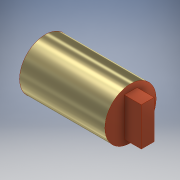
# Autodesk Inventor part: 레이져
Saved by Autodesk Inventor 2018 (Build 220112000, 112)
## iProperties
Created: 2018-04-19
Part Number: 레이져
Material: 일반
Document SubType Name: Modeling
Designer: CK
Density: 1 g/cm^3
Appearance: 금속 1400F 열
Author: CK
Autodesk Inventor part; units mm, degrees
ref_plane "YZ Plane" through (0, 0, 0) normal (1, 0, 0) x (0, 1, 0)
ref_plane "XZ Plane" through (0, 0, 0) normal (0, 1, 0) x (-1, 0, 0)
ref_plane "XY Plane" through (0, 0, 0) normal (0, 0, 1) x (1, 0, 0)
sketch "스케치1" plane through (0, 0, 0) normal (1, 0, 0) x (0, 1, 0)
  circle A0 centre (0, 0) radius 3
  dimension "d0" = 6
  constraints: 1 centre point, 1 coincident
  measures "d0" diameter of A0
extrude "돌출1" add sketch "스케치1" along normal blind 10
sketch "스케치2" plane through (0, 0, 0) normal (-1, 0, 0) x (0, 0, 1)
  circle A0 centre (0, 0) radius 1.5
  dimension "d3" = 3
  constraints: 1 centre point, 1 coincident
  measures "d3" diameter of A0
extrude "돌출2" cut sketch "스케치2" against normal blind 9
sketch "스케치4" plane through (0, 0, 0) normal (-1, 0, 0) x (0, 0, 1)
  arc A0 (-1.5, 0) -> (1.5, 0) centre (0, 0) ccw
  line L0 (-1.5, 0) -> (1.5, 0)
  line L1 (-2.0992, 0) -> (3.7582, 0)
  constraints: 4 end point, 2 horizontal, 2 point on circle, 1 centre point, 1 coincident
revolve "회전1" add sketch "스케치4" angle 360 about axis through (0, 0, -2.0992) along (0, 0, 1)
sketch "스케치5" plane through (10, 0, 0) normal (1, 0, 0) x (0, 0, -1)
  line L0 (2.2555, 0.7646) -> (-2.2445, 0.7646)
  line L1 (-2.2445, 0.7646) -> (-2.2445, -0.7354)
  line L2 (-2.2445, -0.7354) -> (2.2555, -0.7354)
  line L3 (2.2555, -0.7354) -> (2.2555, 0.7646)
  point P0 (0, 0)
  dimension "d8" = 4.5
  dimension "d9" = 1.5
  constraints: 8 end point, 2 parallel, 1 horizontal, 1 perpendicular
  measures "d8" distance of L2.end L1.end
  measures "d9" distance of L1.end L0.end
extrude "돌출3" add sketch "스케치5" along normal blind 2
